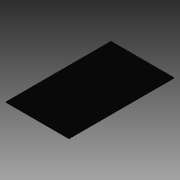
# Autodesk Inventor part: Base Plate
Saved by Autodesk Inventor 2015 (Build 190159000, 159)
## iProperties
Created: 2017-04-23
Part Number: Base Plate
Material: Generic
Document SubType Name: Modeling
Designer: Raghava
Density: 1 g/cm^3
Appearance: Default
Author: Raghava
Autodesk Inventor part; units mm, degrees
ref_plane "YZ Plane" through (0, 0, 0) normal (1, 0, 0) x (0, 1, 0)
ref_plane "XZ Plane" through (0, 0, 0) normal (0, 1, 0) x (-1, 0, 0)
ref_plane "XY Plane" through (0, 0, 0) normal (0, 0, 1) x (1, 0, 0)
sketch "Sketch1" plane through (0, 0, 0) normal (0, 1, 0) x (-1, 0, 0)
  line L0 (-90, 150) -> (90, 150)
  line L1 (90, 150) -> (90, -150)
  line L2 (90, -150) -> (-90, -150)
  line L3 (-90, -150) -> (-90, 150)
  line L4 (-90, 150) -> (90, -150) construction
  line L5 (90, 150) -> (-90, -150) construction
  line L6 (-60, 60) -> (60, 60) construction
  line L7 (60, 60) -> (60, -60) construction
  line L8 (60, -60) -> (-60, -60) construction
  line L9 (-60, -60) -> (-60, 60) construction
  line L10 (-60, 60) -> (60, -60) construction
  line L11 (60, 60) -> (-60, -60) construction
  circle A0 centre (-60, 60) radius 2.5
  circle A1 centre (60, 60) radius 2.5
  circle A2 centre (60, -60) radius 2.5
  circle A3 centre (-60, -60) radius 2.5
  circle A4 centre (60, -137) radius 2.5
  circle A5 centre (-60, -137) radius 2.5
  circle A6 centre (60, 137) radius 2.5
  circle A7 centre (-60, 137) radius 2.5
  point P0 (0, 0)
  dimension "d0" = 180
  dimension "d1" = 300
  dimension "d2" = 120
  dimension "d3" = 120
  dimension "d4" = 5
  dimension "d5" = 5
  dimension "d6" = 5
  dimension "d7" = 5
  dimension "d10" = 5
  dimension "d13" = 120
  dimension "d16" = 274
  dimension "d19" = 13
  dimension "d20" = 30
  constraints: 24 end point, 8 centre point, 4 coincident, 4 midpoint, 4 parallel, 3 horizontal, 2 perpendicular, 1 vertical, 6 other
  measures "d0" distance of L1.end L2.end
  measures "d1" distance of L0.end L1.end
  measures "d2" distance of L7.end L8.end
  measures "d3" distance of L6.end L7.end
  measures "d4" diameter of A0
  measures "d5" diameter of A1
  measures "d6" diameter of A2
  measures "d7" diameter of A3
  measures "d10" diameter of A4
  measures "d13" distance of A4.centre A5.centre
  measures "d16" distance of A4.centre A6.centre
  measures "d19" distance from line of L0 A6.centre
  measures "d20" distance from line of L1 A6.centre
extrude "Extrusion1" add sketch "Sketch1" along normal blind 3
body "Solid2"
